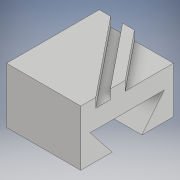
# Autodesk Inventor part: SólidoB
Saved by Autodesk Inventor 2018 (Build 220112000, 112)
## iProperties
Created: 2017-10-07
Part Number: SólidoB
Material: Generic
Document SubType Name: Modeling
Designer: Soichi
Density: 1 g/cm^3
Appearance: Default
Author: Soichi
Autodesk Inventor part; units mm, degrees
ref_plane "YZ Plane" through (0, 0, 0) normal (1, 0, 0) x (0, 1, 0)
ref_plane "XZ Plane" through (0, 0, 0) normal (0, 1, 0) x (-1, 0, 0)
ref_plane "XY Plane" through (0, 0, 0) normal (0, 0, 1) x (1, 0, 0)
sketch "Sketch1" plane through (0, 0, 0) normal (1, 0, 0) x (0, 1, 0)
  line L0 (0, 25) -> (30, 25)
  line L1 (30, 25) -> (30, -25)
  line L2 (30, -25) -> (0, -25)
  line L3 (0, -25) -> (0, 25)
  line L4 (15, 20) -> (15, -20)
  line L5 (0, 0) -> (15, 0) construction
  line L6 (15, 20) -> (0, 8)
  line L7 (15, -20) -> (0, -8)
  line L8 (0, 8) -> (0, -8)
  dimension "d0" = 30
  dimension "d1" = 50
  dimension "d2" = 40
  dimension "d3" = 15
  dimension "d4" = 8
  constraints: 18 end point, 2 horizontal, 2 midpoint, 2 parallel, 1 coincident, 1 collinear, 1 perpendicular, 1 point on line, 1 symmetric about line, 1 vertical
  measures "d0" distance of L1.end L2.end
  measures "d1" distance of L0.end L1.end
  measures "d2" distance of L4.start L4.end
  measures "d3" distance of L5.end L5.start
  measures "d4" distance from line of L6.end L5
extrude "Extrusion1" add sketch "Sketch1" along normal blind 40 contours L0 L1 L2 L3 L7 L4 L6
sketch "Sketch2" plane through (0, 30, 25) normal (0, 1, 0) x (1, 0, 0)
  line L0 (0, 50) -> (40, 50) construction
  line L1 (40, 50) -> (19, 50)
  line L2 (40, 50) -> (40, 24)
  line L3 (40, 33) -> (40, 50) projected
  line L4 (19, 50) -> (40, 24)
  line L5 (45, 9.852) -> (45, 55)
  line L6 (45, 55) -> (8.5343, 55)
  line L7 (8.5343, 55) -> (45, 9.852)
  line L8 (50, -4.296) -> (50, 60)
  line L9 (50, 60) -> (-1.9314, 60)
  line L10 (-1.9314, 60) -> (50, -4.296)
  line L11 (40, 50) -> (40, 0) construction
  point P0 (0, 25)
  dimension "d7" = 21
  dimension "d8" = 26
  dimension "d9" = 5
  dimension "d10" = 5
  constraints: 18 end point, 1 collinear, 1 point on line, 4 other
  measures "d7" distance of L0.end L1.end
  measures "d8" distance of L0.end L2.end
  measures "d9" distance between parallel lines of L4 L7
  measures "d10" distance between parallel lines of L10 L7
extrude "Extrusion2" cut sketch "Sketch2" against normal blind 5
body "Solid1"
